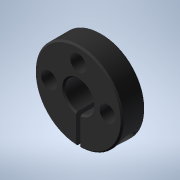
# Autodesk Inventor part: SCST10-8b
Saved by Autodesk Inventor 2021 (Build 250183000, 183)
## iProperties
Created: 2025-09-06
Part Number: SCST10-8b
Material: Generic
Catalog Web Link: www.cadenas.de
Description: SCST, PSCST, SSCST, SCSTR, PSCSTR, SSCSTR-b-Set Collars - Slit 3 Hole/3 Tap - Standard Type -
Vendor: MISUMI
Document SubType Name: Modeling
Designer: psAdmin
Manufacturer: MISUMI
Mass: 4.01959 g
Surface Area: 27.8685 cm^2
Volume: 4.01959 cm^3
Density: 1 g/cm^3
Appearance: PSOLRGB-175-175-175
Category: PARTsolutions
Company: MISUMI
Title: SCST10-8
Author: Cadenas PARTsolutions
Comments: Set Collars - Slit 3 Hole/3 Tap - Standard Type -
PSOL_IDENT_0: {$CADENAS_DATA/23d-libs/misumi/metric/03_set_collars/scst/scst_b.prj},208 {VTYP=3D},{NB=SCST10-8b},{
PSOL_IDENT_1: LINA=SCST10-8},{NN=SCST, PSCST, SSCST, SCSTR, PSCSTR, SSCSTR-b},{DATE=29.11.2024 04:05:20},{GEOMDATE=
PSOL_IDENT_2: 15.09.2021 06:06:07},{VERSION=},{LINEID=60},{WBVAR=TS,MAT,ST,BS},{WBNUMERIC=BS}  {NB=SCST10-8b},{LIN
PSOL_IDENT_3: A=SCST10-8},{KT=DUMMY},{PN=SCST10-8},{TYPE=SCST},{TS=3H},{TSALG= '3H' , '3-Hole' , '3T' , '3-Tapped'
PSOL_IDENT_4: },{TSA='3H', '3-Hole', '3T', '3 Tap (Coarse)'},{MAT=S45C},{ST=BO},{STALG= 'BO' , 'Black Oxide' , 'E
PSOL_IDENT_5: NP' , 'Electroless Nickel Plating' },{AC=Hex Socket Head Cap Screw 1 pc.},{ACMAT=4137 Alloy Steel},{
PSOL_IDENT_6: D=10},{BS=8},{BALG= 8 , 10 , 12 ,15 },{D1=30},{M=M3},{M3D=3},{DD=3.4},{R=3.00},{W=1.5},{X=9.0},{Y=5}
PSOL_IDENT_7: ,{P=20},{C=0.5},{S=5.5},{M1=-},{M13D=0},{L=14}
NB: SCST10-8b
NN: SCST, PSCST, SSCST, SCSTR, PSCSTR, SSCSTR-b
NT: Set Collars - Slit 3 Hole/3 Tap - Standard Type -
NBSYN: $PN.b
LINA: SCST10-8
CATALOG: Misumi
PN: SCST10-8
TS: 3-Hole
MAT: 1045 Carbon Steel
ST: Black Oxide
AC: Hex Socket Head Cap Screw 1 pc.
ACMAT: 4137 Alloy Steel
D: 10
BS: 8
D1: 30
M: M3
DD: 3.4
R: 3
W: 1.5
X: 9
Y: 5
P: 20
C: 0.5
S: 5.5
M1: -
SUPPLIER: MISUMI
ARTICLENO: SCST10-8b
BOMINFO: SCST10-8
CREATOR: CADENAS GmbH
Autodesk Inventor part; units mm, degrees
sketch "Sketch_14" plane through (0, 0, 0) normal (1, 0, 0) x (0, 1, 0)
  line L0 (0, -4) -> (0, 4)
  line L1 (0, 4) -> (14.5, 4)
  line L2 (14.5, 4) -> (15, 3.5)
  line L3 (15, 3.5) -> (15, -3.5)
  line L4 (15, -3.5) -> (14.5, -4)
  line L5 (14.5, -4) -> (0, -4)
  line L6 (0, -4) -> (0, 4)
  constraints: 14 end point
revolve "Revolution1" add sketch "Sketch_14" angle 360 about axis through (0, 0, -4) along (0, 0, -1)
sketch "Sketch_15" plane through (0, 0, 0) normal (1, 0, 0) x (0, 1, 0)
  line L0 (0, -4) -> (0, 4)
  line L1 (0, 4) -> (5.5, 4)
  line L2 (5.5, 4) -> (5, 3.5)
  line L3 (5, 3.5) -> (5, -3.5)
  line L4 (5, -3.5) -> (5.5, -4)
  line L5 (5.5, -4) -> (0, -4)
  line L6 (0, -4) -> (0, 4)
  constraints: 14 end point
revolve "Revolution2" cut sketch "Sketch_15" angle 360 about axis through (0, 0, -4) along (0, 0, -1)
sketch "Sketch_16" plane through (0, 0, 0) normal (0, 0, 1) x (1, 0, 0)
  arc A0 (-0.75, -15.9824) -> (0.75, -15.9824) centre (0, 0) ccw
  line L0 (0.75, -15.9824) -> (0.75, 0)
  line L1 (0.75, 0) -> (-0.75, 0)
  line L2 (-0.75, 0) -> (-0.75, -15.9824)
  constraints: 6 end point, 2 point on circle, 1 centre point
extrude "Extrusion1" cut sketch "Sketch_16" along normal mid plane 8
sketch "Sketch4" plane through (0, 0, -4) normal (0, 0, -1) x (-1, 0, 0)
  point P0 (-10, 0)
hole "Hole1" at (10, 0, -4) direction (0, 0, 1) diameter 5.5 depth 8
sketch "Sketch5" plane through (0, 0, -4) normal (0, 0, -1) x (-1, 0, 0)
  point P0 (10, 0)
hole "Hole2" at (-10, 0, -4) direction (0, 0, 1) diameter 5.5 depth 8
sketch "Sketch6" plane through (0, 0, -4) normal (0, 0, -1) x (-1, 0, 0)
  point P0 (0, 10)
hole "Hole3" at (0, 10, -4) direction (0, 0, 1) diameter 5.5 depth 8
sketch "Sketch_23" plane through (0, -9, 0) normal (0, 1, 0) x (1, 0, 0)
  line L0 (15, 0) -> (0, 0)
  line L1 (0, 0) -> (0, 1.7)
  line L2 (0, 1.7) -> (5, 1.7)
  line L3 (5, 1.7) -> (5, 3)
  line L4 (5, 3) -> (15, 3)
  line L5 (15, 3) -> (15, 0)
  line L6 (15, 0) -> (0, 0)
  constraints: 14 end point
revolve "Revolution3" cut sketch "Sketch_23" angle 360 about axis through (15, -9, 0) along (1, 0, 0)
sketch "Sketch8" plane through (-0.75, -14.4806, 4) normal (1, 0, 0) x (0, 0, -1)
  point P0 (4, 5.4806)
hole "Hole4" at (-0.75, -9, 0) direction (-1, 0, 0) diameter 2.459 depth 12.2404 countersink diameter 3 countersink angle 90 thread size "M3x0.5" class "6H" standard "ISO Metric profile"
ref_plane "to_bolt_XY" through (5, -9, 0) normal (1, 0, 0) x (0, 0, -1)
ref_plane "to_bolt_YZ" through (5, -9, 0) normal (0, 0, -1) x (0, 1, 0)
ref_plane "to_bolt_ZX" through (5, -9, 0) normal (0, 1, 0) x (1, 0, 0)
body "Solid1"
